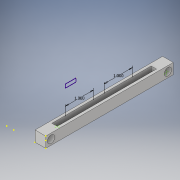
# Autodesk Inventor part: MTV horizantal connector (12.10)
Saved by Autodesk Inventor 2018 (Build 220112000, 112)
## iProperties
Created: 2018-11-26
Part Number: MTV horizantal connector (12.10)
Material: Generic
Document SubType Name: Sheet Metal
Designer: Aditya Kendre
Density: 1 g/cm^3
Appearance: Default
Sheet Metal Rule: Default
Author: Aditya Kendre
## iProperties of the stored document MTV Truning Connecter (11_3DPrint.ipt
Created: 2018-11-27
Part Number: MTV Truning Connecter (11_3DPrint
Material: Generic
Document SubType Name: Modeling
Designer: Aditya Kendre
Density: 1 g/cm^3
Appearance: Default
Author: Aditya Kendre
Autodesk Inventor part; units mm, degrees
ref_plane "YZ Plane" through (0, 0, 0) normal (1, 0, 0) x (0, 1, 0)
ref_plane "XZ Plane" through (0, 0, 0) normal (0, 1, 0) x (-1, 0, 0)
ref_plane "XY Plane" through (0, 0, 0) normal (0, 0, 1) x (1, 0, 0)
sketch "Sketch1" plane through (0, 0, 0) normal (0, 1, 0) x (-1, 0, 0)
  line L0 (0, 0) -> (9.525, 0)
  line L1 (9.525, 0) -> (9.525, -114.3)
  line L2 (9.525, -114.3) -> (0, -114.3)
  line L3 (0, -114.3) -> (0, 0)
  dimension "d0" = 9.525
  dimension "d1" = 114.3
  constraints: 8 end point, 2 parallel, 1 horizontal, 1 perpendicular
  measures "d0" distance of L1.end L2.end
  measures "d1" distance of L0.end L1.end
extrude "Extrusion1" add sketch "Sketch1" along normal blind 9.525
sketch "Sketch2" plane through (0, 9.525, 0) normal (0, 1, 0) x (1, 0, 0)
  point P0 (0, 0)
  point P1 (-2.3813, 12.7)
sketch "Sketch3" plane through (0, 9.525, 0) normal (0, 1, 0) x (1, 0, 0)
  line L0 (-2.3876, 12.7) -> (-7.1501, 12.7)
  line L1 (-7.1501, 12.7) -> (-7.1501, 101.6)
  line L2 (-7.1501, 101.6) -> (-2.3876, 101.6)
  line L3 (-2.3876, 101.6) -> (-2.3876, 12.7)
  point P0 (0, 0)
  dimension "d4" = 4.7625
  dimension "d5" = 88.9
  constraints: 8 end point, 2 parallel, 1 horizontal, 1 perpendicular
  measures "d4" distance of L1.end L2.end
  measures "d5" distance of L0.end L1.end
extrude "Extrusion2" cut sketch "Sketch3" against normal blind 9.525
sketch "Sketch4" plane through (0, 0, 0) normal (1, 0, 0) x (0, 0, -1)
  circle A0 centre (6.1453, 4.7625) radius 3.175
  circle A1 centre (6.1453, 4.7625) radius 3.302
  point P0 (0, 0)
  dimension "d8" = 6.35
  dimension "d9" = 6.604
  constraints: 2 centre point, 1 coincident
  measures "d8" diameter of A0
  measures "d9" diameter of A1
extrude "Extrusion3" cut sketch "Sketch4" against normal blind 8.255 contours A0 | A1
sketch "Sketch5" plane through (0, 0, 0) normal (1, 0, 0) x (0, 0, -1)
  point P0 (0, 0)
  point P1 (107.95, 4.7625)
sketch "Sketch6" plane through (0, 0, 0) normal (1, 0, 0) x (0, 0, -1)
  circle A0 centre (6.1453, 4.7625) radius 3.302 projected
  circle A1 centre (6.1453, 4.7625) radius 3.302
  point P0 (0, 0)
  constraints: 1 centre point, 1 coincident
extrude "Extrusion4" add sketch "Sketch6" against normal blind 9.2075
sketch "Sketch7" plane through (0, 0, 0) normal (1, 0, 0) x (0, 0, -1)
  circle A0 centre (4.7752, 4.7625) radius 3.302
  circle A1 centre (109.5248, 4.7752) radius 3.302
  point P0 (0, 0)
  dimension "d14" = 6.604
  dimension "d15" = 6.604
  constraints: 2 centre point, 1 coincident
  measures "d14" diameter of A0
  measures "d15" diameter of A1
extrude "Extrusion5" cut sketch "Sketch7" against normal blind 7.62
sketch "Sketch8" plane through (-9.525, 0, -114.3) normal (-1, 0, 0) x (0, 0, 1)
  line L0 (61.9125, 3.175) -> (52.3875, 3.175)
  line L1 (52.3875, 3.175) -> (52.3875, 6.35)
  line L2 (52.3875, 6.35) -> (61.9125, 6.35)
  line L3 (61.9125, 6.35) -> (61.9125, 3.175)
  line L4 (61.9125, 3.175) -> (52.3875, 6.35) construction
  line L5 (52.3875, 3.175) -> (61.9125, 6.35) construction
  point P0 (114.3, 0)
  point P1 (57.15, 4.7625)
  dimension "d18" = 9.525
  dimension "d19" = 3.175
  constraints: 12 end point, 2 midpoint, 2 parallel, 1 horizontal, 1 perpendicular
  measures "d18" distance of L1.end L2.end
  measures "d19" distance of L0.end L1.end
extrude "Extrusion6" add sketch "Sketch8" along normal blind 19.05
sketch "Sketch9" plane through (-9.525, 6.35, -52.3875) normal (0, 1, 0) x (1, 0, 0)
  point P0 (9.525, -52.3875)
sketch "Sketch10" plane through (-28.575, 0, -114.3) normal (-1, 0, 0) x (0, 0, 1)
  point P0 (114.3, 0)
sketch "Sketch11" plane through (-28.575, 0, -114.3) normal (-1, 0, 0) x (0, 0, 1)
  line L0 (61.9125, 3.175) -> (52.3875, 3.175) projected
  line L1 (52.3875, 6.35) -> (61.9125, 6.35) projected
  line L2 (52.3875, 3.175) -> (61.9125, 3.175)
  line L3 (61.9125, 3.175) -> (61.9125, 6.35)
  line L4 (61.9125, 6.35) -> (52.3875, 6.35)
  line L5 (52.3875, 6.35) -> (52.3875, 3.175)
  point P0 (114.3, 0)
  constraints: 8 end point, 2 parallel, 1 horizontal, 1 perpendicular
extrude "Extrusion7" add sketch "Sketch11" along normal blind 6.35
sketch "Sketch12" plane through (-34.925, 0, -114.3) normal (-1, 0, 0) x (0, 0, 1)
  line L0 (52.3875, 6.35) -> (61.9125, 6.35) projected
  line L1 (52.3875, 3.175) -> (52.3875, 6.35) projected
  line L2 (61.9125, 6.35) -> (52.3875, 6.35)
  line L3 (52.3875, 6.35) -> (52.3875, 3.175)
  line L4 (52.3875, 3.175) -> (61.9125, 3.175)
  line L5 (61.9125, 3.175) -> (61.9125, 6.35)
  point P0 (114.3, 0)
  constraints: 8 end point, 2 parallel, 1 horizontal, 1 perpendicular
sketch "Sketch13" plane through (-9.525, 3.175, -61.9125) normal (0, -1, 0) x (1, 0, 0)
  circle A0 centre (-20.6248, 4.7625) radius 3.175
  point P0 (9.525, 61.9125)
  dimension "d24" = 6.35
  constraints: 1 centre point
  measures "d24" diameter of A0
extrude "Extrusion8" cut sketch "Sketch13" against normal blind 6.35
fillet "Fillet1" radius 3.175 2 edges at (-9.525, 6.35, -57.15) (-9.525, 3.175, -57.15)
fillet "Fillet2" radius 3.175 2 edges at (-9.525, 4.7625, -52.3875) (-9.525, 4.7625, -61.9125)
sketch "Sketch14" plane through (-9.525, 0, 0) normal (-1, 0, 0) x (0, 0, 1)
  line L0 (-61.9125, 3.175) -> (-52.3875, 3.175) projected
  line L1 (-61.9125, 3.175) -> (-87.3125, 3.175)
  line L2 (-87.3125, 3.175) -> (-87.3125, 6.35)
  line L3 (-87.3125, 6.35) -> (-61.9125, 6.35)
  line L4 (-61.9125, 6.35) -> (-61.9125, 3.175)
  line L5 (-49.2125, 0) -> (-52.3875, 3.175) projected
  line L6 (-52.3875, 3.175) -> (-26.9875, 3.175)
  line L7 (-26.9875, 3.175) -> (-26.9875, 6.35)
  line L8 (-26.9875, 6.35) -> (-52.3875, 6.35)
  line L9 (-52.3875, 6.35) -> (-52.3875, 3.175)
  point P0 (0, 0)
  dimension "d29" = 25.4
  dimension "d30" = 25.4
  constraints: 16 end point, 4 parallel, 2 horizontal, 2 perpendicular, 1 point on line
  measures "d29" distance of L2.end L3.end
  measures "d30" distance of L8.end L7.end
sketch "Sketch15" plane through (-9.525, 0, 0) normal (-1, 0, 0) x (0, 0, 1)
  point P0 (0, 0)
sketch "Sketch16" plane through (-34.925, 6.35, -52.3875) normal (0, 1, 0) x (1, 0, 0)
  arc A0 (25.3996, 34.9251) -> (25.3996, -25.3998) centre (30.609, 4.7627) ccw
  line L0 (25.3996, 34.9251) -> (25.3996, -25.3998)
  line L1 (25.4, 61.9125) -> (25.4, 12.7) projected
  point P0 (34.925, -52.3875)
  constraints: 2 end point, 2 point on circle, 1 centre point, 1 parallel
sketch "Sketch17" plane through (-34.925, 6.35, -52.3875) normal (0, 1, 0) x (1, 0, 0)
  circle A0 centre (4.7752, 4.7625) radius 3.175 projected
  point P0 (34.925, -52.3875)
  constraints: 1 coincident
sketch "Sketch18" plane through (0, 9.525, 0) normal (0, 1, 0) x (1, 0, 0)
  point P0 (0, 0)
sketch "Sketch19" plane through (-9.525, 0, -114.3) normal (-1, 0, 0) x (0, 0, 1)
  point P0 (114.3, 0)
extrude "Extrusion9" add sketch "Sketch16" against normal blind 3.175
hole "Hole1" at (-30.1498, 6.35, -57.15) direction (0, -1, 0) diameter 6.35 depth 3.048 tip angle 118
sketch "Sketch20" plane through (0, 9.525, 0) normal (0, 1, 0) x (1, 0, 0)
  line L0 (-9.525, 0) -> (-9.525, 49.2125) projected
  line L1 (-9.525, 0) -> (-38.3402, 0)
  line L2 (-38.3402, 0) -> (-38.3402, 114.3)
  line L3 (-38.3402, 114.3) -> (-9.525, 114.3)
  line L4 (-9.525, 114.3) -> (-9.525, 0)
  point P0 (0, 0)
  constraints: 8 end point, 2 parallel, 1 horizontal, 1 perpendicular
extrude "Extrusion10" cut sketch "Sketch20" against normal blind 25.4
sketch "Sketch21" plane through (0, 0, 0) normal (1, 0, 0) x (0, 0, -1)
  circle A0 centre (4.7752, 4.7625) radius 3.302 projected
  circle A1 centre (4.7752, 4.7625) radius 3.302
  circle A2 centre (109.5248, 4.7752) radius 3.302 projected
  circle A3 centre (109.5248, 4.7752) radius 3.302
  point P0 (0, 0)
  constraints: 2 centre point, 2 coincident
extrude "Extrusion11" cut sketch "Sketch21" against normal blind 12.7
equation "\"d38\" = Thickness"
equation "\"BendRadius\" = Thickness"
equation "\"BendReliefWidth\" = Thickness"
equation "\"BendReliefDepth\" = 0.5 * Thickness"
equation "\"CornerReliefSize\" = 4 * Thickness"
equation "\"MinimumRemnant\" = 2 * Thickness"
equation "\"TransitionRadius\" = BendRadius"
equation "\"JacobiRadiusSize\" = Thickness"
equation "\"GapSize\" = Thickness"
equation "\"Thickness\" = 3.048"
body "Solid1"
